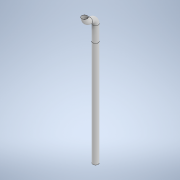
# Autodesk Inventor part: waterpipe3
Saved by Autodesk Inventor 2020 (Build 240168000, 168)
## iProperties
Created: 2019-07-31
Part Number: waterpipe3
Material: Generic
Document SubType Name: Modeling
Designer: ColinP
Density: 1 g/cm^3
Appearance: Default
Author: ColinP
Autodesk Inventor part; units mm, degrees
ref_plane "YZ Plane" through (0, 0, 0) normal (1, 0, 0) x (0, 1, 0)
ref_plane "XZ Plane" through (0, 0, 0) normal (0, 1, 0) x (-1, 0, 0)
ref_plane "XY Plane" through (0, 0, 0) normal (0, 0, 1) x (1, 0, 0)
sketch "Sketch1" plane through (0, 0, 0) normal (0, 1, 0) x (-1, 0, 0)
  circle A0 centre (0, 0) radius 3.175
  circle A1 centre (0, 0) radius 3.048
  dimension "d0" = 6.35
  dimension "d1" = 6.096
  constraints: 2 centre point, 2 coincident
  measures "d0" diameter of A0
  measures "d1" diameter of A1
extrude "Extrusion1" add sketch "Sketch1" along normal blind 121.92
sketch "Sketch8" plane through (0, 0, 0) normal (1, 0, 0) x (0, 1, 0)
  line L0 (121.92, -3.175) -> (121.92, 3.175) projected
  line L1 (121.92, 0) -> (139.7, 0)
  arc A0 (139.7, 0) -> (146.05, 6.35) centre (139.7, 6.35) ccw
  arc A1 (152.4, 12.7) -> (146.05, 6.35) centre (152.4, 6.35) ccw
  point P0 (0, 0)
  dimension "d31" = 17.78
  constraints: 4 point on circle, 2 centre point, 2 end point, 1 midpoint
  measures "d31" distance of L1.start L1.end
sketch "Sketch9" plane through (0, 121.92, 0) normal (0, 1, 0) x (1, 0, 0)
  circle A0 centre (0, 0) radius 3.175 projected
  circle A1 centre (0, 0) radius 3.048 projected
sweep "Sweep4" add profiles "Sketch9" path "Sketch8" separate body path curves L1 A0 A1
body "Solid1"
body "Solid5"
